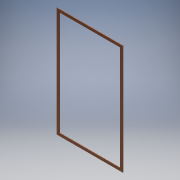
# Autodesk Inventor part: Rahmen 1
Saved by Autodesk Inventor 2017 (Build 210142000, 142)
## iProperties
Created: 2017-05-11
Part Number: Rahmen 1
Material: Holz (Eiche)
Document SubType Name: Modeling
Designer: Fake
Density: 0.76 g/cm^3
Appearance: Weißeiche - natur - mittlerer Glanz
Author: Fake
Autodesk Inventor part; units mm, degrees
ref_plane "YZ Plane" through (0, 0, 0) normal (1, 0, 0) x (0, 1, 0)
ref_plane "XZ Plane" through (0, 0, 0) normal (0, 1, 0) x (-1, 0, 0)
ref_plane "XY Plane" through (0, 0, 0) normal (0, 0, 1) x (1, 0, 0)
sketch "Skizze1" plane through (0, 0, 0) normal (0, 1, 0) x (-1, 0, 0)
  line L0 (600, 1000) -> (-600, 1000)
  line L1 (-600, 1000) -> (-600, -1000)
  line L2 (-600, -1000) -> (600, -1000)
  line L3 (600, -1000) -> (600, 1000)
  line L4 (840, 0) -> (-840, 0) projected
  line L5 (0, -1400) -> (0, 1400) projected
  line L6 (-550, 950) -> (550, 950)
  line L7 (550, 950) -> (550, -950)
  line L8 (550, -950) -> (-550, -950)
  line L9 (-550, -950) -> (-550, 950)
  dimension "d2" = 2000
  dimension "d3" = 1200
  dimension "d4" = 50
  constraints: 16 end point, 4 parallel, 2 perpendicular, 1 horizontal, 5 other
  measures "d2" distance of L2.end L0.start
  measures "d3" distance of L0.start L0.end
  measures "d4" distance between parallel lines of L3 L7
extrude "Extrusion1" add sketch "Skizze1" along normal blind 10 contours L3 L4 L7 L6 L5 L0 | L5 L6 L9 L4 L1 L0 | L3 L2 L5 L8 L7 L4 | L4 L9 L8 L5 L2 L1
